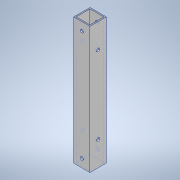
# Autodesk Inventor part: ロボットベース15x15_4
Saved by Autodesk Inventor 2020.3 (Build 243373000, 373)
## iProperties
Created: 2020-07-04
Part Number: ロボットベース15x15_4
Material: アルミニウム 6061
Document SubType Name: Modeling
Designer: totot
Density: 2.7 g/cm^3
Appearance: アルミニウム - フラット
Author: totot
Autodesk Inventor part; units mm, degrees
ref_plane "YZ Plane" through (0, 0, 0) normal (1, 0, 0) x (0, 1, 0)
ref_plane "XZ Plane" through (0, 0, 0) normal (0, 1, 0) x (-1, 0, 0)
ref_plane "XY Plane" through (0, 0, 0) normal (0, 0, 1) x (1, 0, 0)
sketch "スケッチ1" plane through (0, 0, 0) normal (0, 1, 0) x (-1, 0, 0)
  line L0 (0, 0) -> (-15, 0)
  line L1 (-15, 0) -> (-15, 15)
  line L2 (-15, 15) -> (0, 15)
  line L3 (0, 15) -> (0, 0)
  line L4 (-1.2, 13.8) -> (-13.8, 13.8)
  line L5 (-13.8, 13.8) -> (-13.8, 1.2)
  line L6 (-13.8, 1.2) -> (-1.2, 1.2)
  line L7 (-1.2, 1.2) -> (-1.2, 13.8)
  dimension "d0" = 15
  dimension "d1" = 15
  dimension "d2" = 1.2
  dimension "d3" = 1.2
  dimension "d4" = 1.2
  dimension "d5" = 1.2
  constraints: 16 end point, 4 parallel, 2 horizontal, 2 perpendicular
  measures "d0" distance of L1.end L2.end
  measures "d1" distance of L0.end L1.end
  measures "d2" distance between parallel lines of L2 L4
  measures "d3" distance between parallel lines of L0 L6
  measures "d4" distance between parallel lines of L7 L3
  measures "d5" distance between parallel lines of L1 L5
extrude "押し出し1" add sketch "スケッチ1" along normal blind 116
sketch "スケッチ2" plane through (0, 0, 15) normal (0, 0, 1) x (1, 0, 0)
  line L0 (0, 116) -> (15, 116) projected
  line L1 (0, 0) -> (15, 0) projected
  line L2 (15, 0) -> (15, 116) projected
  point P0 (7.5, 108.5)
  point P1 (7.5, 7.5)
  dimension "d8" = 7.5
  dimension "d9" = 7.5
  dimension "d10" = 7.5
  dimension "d11" = 7.5
  measures "d8" distance from line of point (7.5, 108.5) L0
  measures "d9" distance from line of L1 point (7.5, 7.5)
  measures "d10" distance from line of point (7.5, 108.5) L2
  measures "d11" distance from line of L2 point (7.5, 7.5)
hole "穴1" at (7.5, 108.5, 15) at (7.5, 7.5, 15) direction (0, 0, -1) diameter 3 end through all
sketch "スケッチ3" plane through (15, 0, 15) normal (1, 0, 0) x (0, 0, -1)
  line L0 (0, 0) -> (15, 0) projected
  line L1 (0, 0) -> (0, 116) projected
  line L2 (0, 116) -> (15, 116) projected
  point P0 (7.5, 22.5)
  point P1 (7.5, 93.5)
  dimension "d19" = 22.5
  dimension "d20" = 7.5
  dimension "d21" = 7.5
  dimension "d22" = 22.5
  measures "d19" distance from line of L0 point (7.5, 22.5)
  measures "d20" distance from line of L1 point (7.5, 22.5)
  measures "d21" distance from line of L1 point (7.5, 93.5)
  measures "d22" distance from line of point (7.5, 93.5) L2
hole "穴2" at (15, 22.5, 7.5) at (15, 93.5, 7.5) direction (-1, 0, 0) diameter 3 end through all
sketch "スケッチ4" plane through (15, 0, 0) normal (0, 0, -1) x (-1, 0, 0)
  line L0 (0, 116) -> (15, 116) projected
  line L1 (0, 0) -> (15, 0) projected
  line L2 (0, 0) -> (0, 116) projected
  point P0 (7.5, 58)
  dimension "d30" = 116
  dimension "d31" = 58
  dimension "d32" = 7.5
  measures "d30" distance between parallel lines of L0 L1
  measures "d31" distance from line of point (7.5, 58) L1
  measures "d32" distance from line of point (7.5, 58) L2
hole "穴3" at (7.5, 58, 0) direction (0, 0, 1) diameter 5 end through all
equation "\"d3\" = d2"
equation "\"d4\" = d2"
equation "\"d5\" = d2"
equation "\"d9\" = d8"
equation "\"d10\" = d8"
equation "\"d11\" = d9"
equation "\"d31\" = 0.5 * d30"
